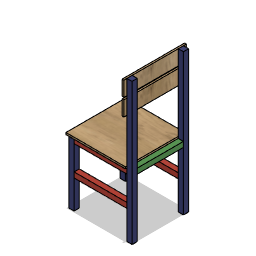
chair v7 (Autodesk Fusion 360 design; units mm, degrees)
Autodesk Fusion 360 part; units mm, degrees
note: some values were not read from the file. Chosen so that the rebuilt part matches the saved one: which bodies a step acts on; which face or edge a step refers to; that a step has no effect.
sketch "スケッチ1" plane through (0, 0, 0) normal (0, 1, 0) x (1, 0, 0)
  line L0 (-190, 190) -> (190, 190)
  line L1 (190, 190) -> (190, -190)
  line L2 (190, -190) -> (-190, -190)
  line L3 (-190, -190) -> (-190, 190)
  line L4 (-190, 190) -> (190, -190) construction
  line L5 (190, 190) -> (-190, -190) construction
  line L6 (-190, 190) -> (-155, 190)
  line L7 (-155, 190) -> (-155, 155)
  line L8 (-155, 155) -> (-190, 155)
  line L9 (-190, 155) -> (-190, 190)
  line L10 (-190, -190) -> (-155, -190)
  line L11 (-155, -190) -> (-155, -155)
  line L12 (-155, -155) -> (-190, -155)
  line L13 (-190, -155) -> (-190, -190)
  line L14 (190, 190) -> (200, 190)
  line L15 (200, 190) -> (200, -190)
  line L16 (200, -190) -> (190, -190)
  line L17 (190, -190) -> (190, 190)
  line L18 (200, 190) -> (235, 190)
  line L19 (235, 190) -> (235, 155)
  line L20 (235, 155) -> (200, 155)
  line L21 (200, 155) -> (200, 190)
  line L22 (200, -190) -> (235, -190)
  line L23 (235, -190) -> (235, -155)
  line L24 (235, -155) -> (200, -155)
  line L25 (200, -155) -> (200, -190)
  dimension "d1" = 380
  dimension "d2" = 380
  dimension "d3" = 35
  dimension "d4" = 35
  dimension "d5" = 35
  dimension "d6" = 35
  dimension "d7" = 10
  dimension "d8" = 380
  dimension "d9" = 35
  dimension "d10" = 35
  dimension "d11" = 35
  dimension "d12" = 35
  constraint perpendicular L0 L1
  constraint parallel L0 L2
  constraint parallel L1 L3
  constraint horizontal L0
  constraint coincident L4 origin
  constraint coincident L5 origin
  constraint horizontal L6
  constraint vertical L7
  constraint horizontal L8
  constraint vertical L9
  constraint horizontal L10
  constraint vertical L11
  constraint horizontal L12
  constraint vertical L13
  constraint horizontal L14
  constraint vertical L15
  constraint horizontal L16
  constraint vertical L17
  constraint horizontal L18
  constraint vertical L19
  constraint horizontal L20
  constraint vertical L21
  constraint horizontal L22
  constraint vertical L23
  constraint horizontal L24
  constraint vertical L25
  measures "d1" distance of L1.end L2.end
  measures "d2" distance of L0.end L1.end
  measures "d3" distance of L0.start L6.end
  measures "d4" distance of L0.start L8.end
  measures "d5" distance of L2.end L10.end
  measures "d6" distance of L2.end L12.end
  measures "d7" distance of L0.end L14.end
  measures "d8" distance of L0.end L1.end
  measures "d9" distance of L14.end L18.end
  measures "d10" distance of L14.end L20.end
  measures "d11" distance of L15.end L22.end
  measures "d12" distance of L15.end L24.end
extrude "押し出し1" add sketch "スケッチ1" along normal blind 428 contours L0 L3 L6 L7 L8 L9 | L2 L3 L10 L11 L12 L13 | L15 L18 L19 L20 L21 | L15 L22 L23 L24 L25 makes body 1 at (211.6667, 142.6667, -190) makes body 2 at (-166.6667, 142.6667, 155) makes body 3 at (-178.3333, 142.6667, -190) makes body 4 at (200, 142.6667, 166.6667)
sketch "スケッチ2" plane through (0, 428, 0) normal (0, 1, 0) x (-1, 0, 0)
  line L0 (-200, -155) -> (-235, -155)
  line L1 (-235, -155) -> (-235, -190)
  line L2 (-235, -190) -> (-200, -190)
  line L3 (-200, -190) -> (-200, -155)
  line L4 (-200, -190) -> (200, -190)
  line L5 (200, -190) -> (200, -200)
  line L6 (200, -200) -> (-200, -200)
  line L7 (-200, -200) -> (-200, -190)
  line L8 (200, -190) -> (-200, -190)
  line L9 (-200, -190) -> (-200, 200)
  line L10 (-200, 200) -> (200, 200)
  line L11 (200, 200) -> (200, -190)
  dimension "d15" = 10
  dimension "d16" = 400
  dimension "d17" = 400
  dimension "d18" = 390
  constraint horizontal L4
  constraint vertical L5
  constraint horizontal L6
  constraint vertical L7
  constraint coincident L2.end L3.start
  constraint horizontal L8
  constraint vertical L9
  constraint horizontal L10
  constraint vertical L11
  measures "d15" distance of L2.end L6.end
  measures "d16" distance of L2.end L4.end
  measures "d17" distance of L4.end L2.end
  measures "d18" distance of L4.end L10.end
extrude "押し出し2" add sketch "スケッチ2" along normal blind 12 separate body contours L3 L4 L8 L9 L10 L11 | L4 L5 L6 L7 L8 makes body 5
sketch "スケッチ3" plane through (200, 0, 0) normal (-1, 0, 0) x (0, 0, 1)
  line L0 (155, 0) -> (190, 0)
  line L1 (190, 0) -> (190, 428)
  line L2 (190, 428) -> (155, 428)
  line L3 (155, 428) -> (155, 0)
  line L4 (190, 428) -> (155, 428)
  line L5 (155, 428) -> (155, 393)
  line L6 (155, 393) -> (190, 393)
  line L7 (190, 393) -> (190, 428)
  dimension "d21" = 35
  constraint horizontal L4
  constraint vertical L5
  constraint horizontal L6
  constraint vertical L7
  constraint coincident L1.end L2.start
  measures "d21" distance of L1.end L6.end
sketch "スケッチ4" plane through (200, 0, 0) normal (-1, 0, 0) x (0, 0, 1)
  line L0 (-190, 0) -> (-155, 0)
  line L1 (-155, 0) -> (-155, 428)
  line L2 (-155, 428) -> (-190, 428)
  line L3 (-190, 428) -> (-190, 0)
  line L4 (-190, 428) -> (-155, 428)
  line L5 (-155, 428) -> (-155, 393)
  line L6 (-155, 393) -> (-190, 393)
  line L7 (-190, 393) -> (-190, 428)
  dimension "d22" = 35
  dimension "d23" = 35
  constraint horizontal L4
  constraint vertical L5
  constraint horizontal L6
  constraint vertical L7
  constraint coincident L2.end L3.start
  measures "d22" distance of L2.end L1.end
  measures "d23" distance of L2.end L6.end
sketch "スケッチ5" plane through (0, 0, 155) normal (0, 0, -1) x (-1, 0, 0)
  line L0 (155, 0) -> (190, 0)
  line L1 (190, 0) -> (190, 428)
  line L2 (190, 428) -> (155, 428)
  line L3 (155, 428) -> (155, 0)
  line L4 (155, 428) -> (190, 428)
  line L5 (190, 428) -> (190, 393)
  line L6 (190, 393) -> (155, 393)
  line L7 (155, 393) -> (155, 428)
  dimension "d24" = 35
  dimension "d25" = 35
  constraint horizontal L4
  constraint vertical L5
  constraint horizontal L6
  constraint vertical L7
  constraint coincident L2.end L3.start
  measures "d24" distance of L2.end L1.end
  measures "d25" distance of L2.end L6.end
extrude "押し出し3" add sketch "スケッチ3" sketch "スケッチ4" along normal blind 355 separate body contours L1 L2 L3 L4 L5 L6 L7 of sketch 2 contours L1 L2 L3 L4 L5 L6 L7 makes body 6 at (81.6667, 416.3333, 155) makes body 7 at (81.6667, 416.3333, -190)
extrude "押し出し4" add sketch "スケッチ5" along normal blind 310 separate body contours L1 L2 L3 L4 L5 L6 L7 makes body 8
sketch "スケッチ6" plane through (0, 0, -155) normal (0, 0, 1) x (1, 0, 0)
  line L0 (200, 393) -> (200, 428)
  line L1 (200, 428) -> (-155, 428)
  line L2 (-155, 428) -> (-155, 393)
  line L3 (-155, 393) -> (200, 393)
  line L4 (200, 428) -> (165, 428)
  line L5 (165, 428) -> (165, 393)
  line L6 (165, 393) -> (200, 393)
  line L7 (200, 393) -> (200, 428)
  dimension "d30" = 35
  constraint horizontal L4
  constraint vertical L5
  constraint horizontal L6
  constraint vertical L7
  constraint coincident L0.end L1.start
  measures "d30" distance of L0.end L4.end
extrude "押し出し5" add sketch "スケッチ6" along normal blind 310 separate body contours L0 L1 L3 L4 L5 L6 L7 makes body 9
sketch "スケッチ7" plane through (0, 0, -155) normal (0, 0, 1) x (1, 0, 0)
  line L0 (200, 0) -> (235, 0)
  line L1 (235, 0) -> (235, 428)
  line L2 (235, 428) -> (200, 428)
  line L3 (200, 428) -> (200, 0)
  line L4 (235, 428) -> (200, 428)
  line L5 (200, 428) -> (200, 393)
  line L6 (200, 393) -> (235, 393)
  line L7 (235, 393) -> (235, 428)
  dimension "d33" = 35
  constraint horizontal L4
  constraint vertical L5
  constraint horizontal L6
  constraint vertical L7
  constraint coincident L1.end L2.start
  measures "d33" distance of L1.end L6.end
extrude "押し出し6" add sketch "スケッチ7" along normal blind 310 separate body contours L1 L2 L3 L4 L5 L6 L7 makes body 10
extrude "押し出し7" add 2 faces at (211.6667, 428, -178.3333) (211.6667, 428, 166.6667) along direction (0, 1, 0) blind 300 on bodies 1 4 bodies 1 8 4 5 6 7 9 10
extrude "押し出し8" add 2 faces at (211.6667, 728, -178.3333) (211.6667, 728, 166.6667) along direction (0, 1, 0) blind 50 on bodies 1 bodies 1
sketch "スケッチ8" plane through (200, 0, 0) normal (-1, 0, 0) x (0, 0, 1)
  line L0 (155, 440) -> (190, 440)
  line L1 (190, 440) -> (190, 778)
  line L2 (190, 778) -> (155, 778)
  line L3 (155, 778) -> (155, 440)
  line L4 (190, 778) -> (210, 778)
  line L5 (210, 778) -> (210, 708)
  line L6 (210, 708) -> (190, 708)
  line L7 (190, 708) -> (190, 778)
  line L8 (190, 778) -> (-210, 778)
  line L9 (-210, 778) -> (-210, 708)
  line L10 (-210, 708) -> (190, 708)
  line L11 (190, 708) -> (190, 778)
  line L12 (-210, 708) -> (210, 708)
  line L13 (210, 708) -> (210, 678)
  line L14 (210, 678) -> (-210, 678)
  line L15 (-210, 678) -> (-210, 708)
  dimension "d40" = 70
  dimension "d41" = 70
  dimension "d42" = 30
  constraint horizontal L4
  constraint vertical L5
  constraint horizontal L6
  constraint vertical L7
  constraint coincident L1.end L2.start
  constraint horizontal L8
  constraint vertical L9
  constraint horizontal L10
  constraint vertical L11
  constraint horizontal L12
  constraint vertical L13
  constraint horizontal L14
  constraint vertical L15
  measures "d40" distance of L1.end L6.end
  measures "d41" distance of L1.end L6.end
  measures "d42" distance of L9.end L14.end
extrude "押し出し9" add sketch "スケッチ8" along normal blind 12 separate body contours L3 L10 L12 L14 L15 | L1 L3 L10 L12 L14 | L1 L6 L12 L13 L14 | L3 L8 L9 L10 L12 | L1 L2 L3 L7 L8 L10 L11 L12 | L1 L4 L5 L6 L7 L11 L12 makes body 11
sketch "スケッチ9" plane through (200, 0, 0) normal (-1, 0, 0) x (0, 0, 1)
  line L0 (-190, 440) -> (-155, 440)
  line L1 (-155, 440) -> (-155, 778)
  line L2 (-155, 778) -> (-190, 778)
  line L3 (-190, 778) -> (-190, 440)
  line L4 (-190, 677.7582) -> (-155, 677.7582)
  line L5 (-155, 677.7582) -> (-155, 662.7582)
  line L6 (-155, 662.7582) -> (-190, 662.7582)
  line L7 (-190, 662.7582) -> (-190, 677.7582)
  line L8 (-190, 662.7582) -> (-210, 662.7582)
  line L9 (-210, 662.7582) -> (-210, 562.7582)
  line L10 (-210, 562.7582) -> (-190, 562.7582)
  line L11 (-190, 562.7582) -> (-190, 662.7582)
  line L12 (-190, 662.7582) -> (210, 662.7582)
  line L13 (210, 662.7582) -> (210, 562.7582)
  line L14 (210, 562.7582) -> (-190, 562.7582)
  line L15 (-190, 562.7582) -> (-190, 662.7582)
  dimension "d45" = 15
  dimension "d46" = 100
  dimension "d47" = 100
  constraint horizontal L4
  constraint vertical L5
  constraint horizontal L6
  constraint vertical L7
  constraint coincident L3 L4.start
  constraint horizontal L8
  constraint vertical L9
  constraint horizontal L10
  constraint vertical L11
  constraint horizontal L12
  constraint vertical L13
  constraint horizontal L14
  constraint vertical L15
  measures "d45" distance of L4.start L6.end
  measures "d46" distance of L6.end L10.end
  measures "d47" distance of L6.end L10.end
extrude "押し出し10" add sketch "スケッチ9" along normal blind 12 separate body contours L3 L8 L9 L10 L11 L15 | L1 L3 L6 L11 L12 L14 L15 | L1 L12 L13 L14 makes body 12
extrude "押し出し11" add 2 faces at (211.6667, 778, -178.3333) (211.6667, 778, 166.6667) along direction (0, 1, 0) blind 250 on bodies 1 bodies 1 11
sketch "スケッチ10" plane through (200, 0, 0) normal (1, 0, 0) x (0, 0, -1)
  line L0 (-190, 678) -> (-190, 778)
  line L1 (-190, 778) -> (-210, 778)
  line L2 (-210, 778) -> (-210, 678)
  line L3 (-210, 678) -> (-190, 678)
  line L4 (-190, 778) -> (-155, 778)
  line L5 (-155, 778) -> (-155, 678)
  line L6 (-155, 678) -> (-190, 678)
  line L7 (-190, 678) -> (-190, 778)
  dimension "d52" = 35
  dimension "d53" = 100
  constraint horizontal L4
  constraint vertical L5
  constraint horizontal L6
  constraint vertical L7
  constraint coincident L0.end L1.start
  measures "d52" distance of L0.end L4.end
  measures "d53" distance of L0.end L0.start
sketch "スケッチ11" plane through (200, 0, 0) normal (1, 0, 0) x (0, 0, -1)
  line L0 (-155, 778) -> (-155, 678)
  line L1 (-155, 678) -> (155, 678)
  line L2 (155, 678) -> (155, 778)
  line L3 (155, 778) -> (-155, 778)
  line L4 (155, 778) -> (190, 778)
  line L5 (190, 778) -> (190, 678)
  line L6 (190, 678) -> (155, 678)
  line L7 (155, 678) -> (155, 778)
  dimension "d54" = 100
  constraint horizontal L4
  constraint vertical L5
  constraint horizontal L6
  constraint vertical L7
  constraint coincident L2.end L3.start
  measures "d54" distance of L2.end L1.end
sketch "スケッチ12" plane through (0, 428, 0) normal (0, 1, 0) x (-1, 0, 0)
  line L0 (-235, -155) -> (-200, -155)
  line L1 (-200, -155) -> (-200, 155)
  line L2 (-200, 155) -> (-235, 155)
  line L3 (-235, 155) -> (-235, -155)
  line L4 (-235, 155) -> (-200, 155)
  line L5 (-200, 155) -> (-200, 190)
  line L6 (-200, 190) -> (-235, 190)
  line L7 (-235, 190) -> (-235, 155)
  line L8 (-235, 190) -> (-200, 190)
  line L9 (-200, 190) -> (-200, -190)
  line L10 (-200, -190) -> (-235, -190)
  line L11 (-235, -190) -> (-235, 190)
  dimension "d55" = 35
  dimension "d56" = 380
  dimension "d57" = 35
  constraint horizontal L4
  constraint vertical L5
  constraint horizontal L6
  constraint vertical L7
  constraint coincident L2.end L3.start
  constraint horizontal L8
  constraint vertical L9
  constraint horizontal L10
  constraint vertical L11
  measures "d55" distance of L2.end L6.end
  measures "d56" distance of L6.end L10.end
  measures "d57" distance of L6.end L5.end
move_body "移動1" bodies 12 1 to x (1, 0, 0) y (0, 1, 0) z (0, 0, 1) at (0, 75, 0)
move_body "移動2" bodies 1 12 to x (1, 0, 0) y (0, 1, 0) z (0, 0, 1) at (0, 125, 0)
move_body "移動3" bodies 12 1 to x (1, 0, 0) y (0, 1, 0) z (0, 0, 1) at (0, 150, 0)
split "分割2" by plane through (200, 350, 155) normal (-1, 0, 0) bodies 1 makes body 13 at (188, 1061.3333, 70) makes body 14 at (-66.6667, 790, -51.6667)
split "分割4" by plane through (0, 778, 0) normal (0, -1, 0) bodies 14 makes body 15 at (70, 743, 178.3333)
split "分割5" by plane through (235, 778, -155) normal (0, 0, 1) and through (235, 778, 155) normal (0, 0, -1) bodies 1 makes body 16 at (223.3333, 823.6667, 190) makes body 17 at (200, 766.3333, -51.6667)
split "分割6" by plane through (200, 743, -155) normal (0, 0, 1) and through (200, 778, 155) normal (0, 0, -1) bodies 15 makes body 18 at (70, 743, 178.3333) makes body 19 at (200, 766.3333, -51.6667)
move_body "移動4" bodies 13 16 19 17 18 1 15 12 14 to x (1, 0, 0) y (0, 1, 0) z (0, 0, 1) at (0, -350, 0)
move_body "移動5" bodies 12 13 to x (1, 0, 0) y (0, 1, 0) z (0, 0, 1) at (0, 200, 0)
copy_body "ボディのコピーと貼り付け1" bodies 15 makes body 20
move_body "移動6" bodies 20 to x (1, 0, 0) y (0, 1, 0) z (0, 0, 1) at (0, -200, 0)
copy_body "ボディのコピーと貼り付け2" bodies 18 makes body 21
move_body "移動7" bodies 21 to x (1, 0, 0) y (0, 1, 0) z (0, 0, 1) at (0, -200, 0)
form "フォーム1" [no effect]
extrude "押し出し12" cut 1 faces at (211.6667, 1028, -178.3333) along direction (0, -1, 0) blind 78 on bodies 1 bodies 1
extrude "押し出し13" cut 1 faces at (211.6667, 1028, 166.6667) along direction (0, -1, 0) blind 78 on bodies 16 bodies 16
move_body "移動8" bodies 13 12 to x (1, 0, 0) y (0, 1, 0) z (0, 0, 1) at (0, -50, 0)
move_body "移動9" bodies 12 13 to x (1, 0, 0) y (0, 1, 0) z (0, 0, 1) at (0, 22, 0)
named bodies: "後ろ脚1", "前脚1", "前脚2", "横1", "背板2", "背板1", "天板", "縦1", "後ろ脚2", "横3", "縦2", "横2", "縦1 (1)", "縦2 (1)"
